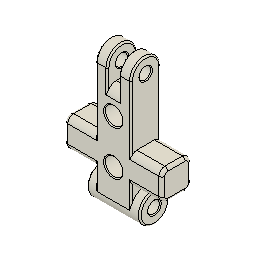
3d-rudder (Autodesk Fusion 360 archive; units mm, degrees)
design "ロードセル固定具"
Autodesk Fusion 360 part; units mm, degrees
sketch "スケッチ1" plane through (0, 0, 0) normal (1, 0, 0) x (0, 0, -1)
  circle A0 centre (0, 0) radius 2
  line L0 (-10, 0) -> (-10, 2)
  line L1 (-10, 2) -> (-11, 2)
  line L2 (-11, 2) -> (-11, 7)
  line L3 (-11, 7) -> (-10, 7)
  line L4 (-10, 7) -> (-10, 13)
  line L5 (-10, 13) -> (-11, 13)
  line L6 (-10, 10) -> (-13, 10)
  line L7 (-13, 10) -> (-13, 25)
  line L8 (-13, 25) -> (-10, 25)
  line L9 (-11, 22) -> (-10, 22)
  line L10 (-10, 22) -> (-10, 28)
  line L11 (-10, 28) -> (-11, 28)
  line L12 (-11, 28) -> (-11, 33)
  line L13 (-11, 33) -> (-10, 33)
  line L14 (-10, 33) -> (-10, 35)
  line L15 (-5, 35) -> (-5, 0)
  line L16 (5, 35) -> (5, 0)
  arc A1 (-5, 0) -> (5, 0) centre (0, 0) ccw
  line L17 (0, 33) -> (0, 38)
  circle A2 centre (0, 38) radius 2
  line L18 (-5, 35) -> (-5, 38)
  line L19 (5, 35) -> (5, 38)
  arc A3 (5, 38) -> (-5, 38) centre (0, 38) ccw
  circle A4 centre (0, 0) radius 5
  dimension "d1" = 4
  dimension "d2" = 15
  constraint coincident A0.centre A1.centre
  constraint vertical L0
  constraint perpendicular L0 L1
  constraint perpendicular L1 L2
  constraint perpendicular L2 L3
  constraint perpendicular L3 L4
  constraint perpendicular L4 L5
  constraint midpoint L4 L6.start
  constraint perpendicular L4 L6
  constraint perpendicular L6 L7
  constraint perpendicular L7 L8
  constraint horizontal L9
  constraint perpendicular L8 L10
  constraint perpendicular L10 L11
  constraint perpendicular L11 L12
  constraint perpendicular L12 L13
  constraint perpendicular L13 L14
  constraint concentric A0 A1
  constraint tangent L15 A1
  constraint vertical L15
  constraint tangent L16 A1
  constraint vertical L16
  constraint parallel L15 L17
  constraint coincident L17.end A2.centre
  constraint concentric A2 A3
  constraint tangent L18 A3
  constraint parallel L15 L18
  constraint tangent L19 A3
  constraint parallel L16 L19
  constraint coincident L15.end A4
  measures "d1" diameter of A0
  measures "d2" distance of L6.end L7.end
extrude "押し出し1" add sketch "スケッチ1" along normal mid plane 12
sketch "スケッチ2" plane through (0, 0, 0) normal (0, 0, 1) x (1, 0, 0)
  line L0 (-15, 2) -> (-15, 7)
  line L1 (-15, 7) -> (-14, 7)
  line L2 (-14, 7) -> (-14, 13)
  line L3 (-14, 13) -> (-15, 13)
  line L4 (-15, 10) -> (-16, 10)
  line L5 (-16, 10) -> (-16, 25)
  line L6 (-16, 25) -> (-15, 25)
  line L7 (-15, 22) -> (-14, 22)
  line L8 (-14, 22) -> (-14, 28)
  line L9 (-14, 28) -> (-15, 28)
  line L10 (-15, 28) -> (-15, 33)
  line L11 (-15, 33) -> (-14, 33)
  line L12 (-14, 33) -> (-14, 35)
  circle A0 centre (0, 25) radius 3
  circle A1 centre (0, 10) radius 3
  dimension "d5" = 15
  dimension "d6" = 6
  dimension "d7" = 6
  constraint vertical L0
  constraint perpendicular L0 L1
  constraint perpendicular L1 L2
  constraint perpendicular L2 L3
  constraint perpendicular L2 L4
  constraint perpendicular L4 L5
  constraint perpendicular L5 L6
  constraint horizontal L7
  constraint perpendicular L7 L8
  constraint perpendicular L8 L9
  constraint perpendicular L9 L10
  constraint perpendicular L8 L11
  constraint perpendicular L11 L12
  measures "d5" distance of L4.end L5.end
  measures "d6" diameter of A0
  measures "d7" diameter of A1
extrude "押し出し2" cut sketch "スケッチ2" along normal mid plane 16
sketch "スケッチ3" plane through (6, 0, 0) normal (1, 0, 0) x (0, 0, -1)
  circle A0 centre (0, 0) radius 2
  line L0 (-5, 38) -> (-5, 0)
  arc A1 (-5, 0) -> (5, 0) centre (0, 0) ccw
  line L1 (5, 0) -> (5, 38)
  arc A2 (5, 38) -> (-5, 38) centre (0, 38) ccw
  circle A3 centre (0, 38) radius 2
  line L2 (-5, 33) -> (5, 33)
  line L3 (0, 38) -> (0, 33)
  line L4 (-3, 7) -> (3, 7)
  line L5 (5, 9) -> (5, 15)
  line L6 (-3, 17) -> (3, 17)
  line L7 (-5, 15) -> (-5, 9)
  arc A4 (-3, 17) -> (-5, 15) centre (-3, 15) ccw
  arc A5 (5, 15) -> (3, 17) centre (3, 15) ccw
  arc A6 (-5, 9) -> (-3, 7) centre (-3, 9) ccw
  arc A7 (3, 7) -> (5, 9) centre (3, 9) ccw
  dimension "d17" = 2
  dimension "d18" = 2
  dimension "d19" = 2
  dimension "d20" = 2
  constraint coincident L0 L2.start
  constraint coincident L1 L2.end
  constraint perpendicular L1 L2
  constraint coincident A2.centre A3.centre
  constraint vertical L3
  constraint perpendicular L1 L4
  constraint perpendicular L1 L6
  constraint tangent L6 A4
  constraint tangent L7 A4
  constraint tangent L6 A5
  constraint tangent L5 A5
  constraint tangent L7 A6
  constraint tangent L4 A6
  constraint tangent L4 A7
  constraint tangent L5 A7
  measures "d17" radius of A4
  measures "d18" radius of A5
  measures "d19" radius of A6
  measures "d20" radius of A7
extrude "押し出し3" cut sketch "スケッチ3" along normal mid plane 4 from surface at -6 contours L0 L1 A2 L2
fillet "フィレット1" radius 3 2 edges at (0, 33, 5) (0, 33, -5)
extrude "押し出し4" add sketch "スケッチ1" along normal mid plane 18 contours A1 A4
extrude "押し出し5" add sketch "スケッチ3" along normal blind 10.5 contours L0 L1 L4 L5 L6 L7 A4 A5 A6 A7
extrude "押し出し6" add sketch "スケッチ3" against normal blind 10.5 from surface at -12 contours L0 L1 L4 L5 L6 L7 A4 A5 A6 A7
fillet "フィレット3" radius 0.5 8 edges at (-2, 34, 5) (-2, 43, 0) (-2, 34, -5) (2, 34, -5) (2, 43, 0) (2, 34, 5) (-6, 4.5, -5) (6, 4.5, -5)
fillet "フィレット4" radius 0.5 2 edges at (9, -1.8081, 4.6616) (-9, 1.8081, 4.6616)
fillet "フィレット5" radius 0.3 10 edges at (-9, -0.7232, 1.8647) (-2.797, 11.0848, 5) (-2.797, 26.0848, 5) (-2.797, 23.9152, -5) (-2.797, 8.9152, -5) (9, 0.7232, 1.8647) (6, 38.7232, 1.8647) (2, 38.7232, 1.8647) (-2, 37.2768, 1.8647) (-6, 37.2768, 1.8647)
fillet "フィレット6" radius 0.5 8 edges at (6, 26.5, -5) (6, 43, 0) (6, 26.5, 5) (-6, 26.5, 5) (-6, 43, 0) (-6, 26.5, -5) (6, 4.5, 5) (-6, 4.5, 5)
fillet "フィレット7" radius 1 16 edges at (16.5, 12, 5) (16.5, 7.5858, 4.4142) (16.5, 7, 0) (16.5, 7.5858, -4.4142) (16.5, 12, -5) (16.5, 16.4142, -4.4142) (16.5, 17, 0) (16.5, 16.4142, 4.4142) (-16.5, 17, 0) (-16.5, 16.4142, -4.4142) (-16.5, 12, -5) (-16.5, 7.5858, -4.4142) (-16.5, 7, 0) (-16.5, 7.5858, 4.4142) (-16.5, 12, 5) (-16.5, 16.4142, 4.4142)
named bodies: "ロードセル固定具LR共通"
